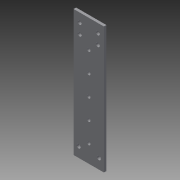
# Autodesk Inventor part: Support for 9-16 Piston
Saved by Autodesk Inventor 2014 (Build 180170000, 170)
## iProperties
Created: 2014-01-07
Part Number: Support for 9-16 Piston
Material: Generic
Document SubType Name: Modeling
Designer: Michael
Density: 1 g/cm^3
Appearance: Default
Author: Michael
Autodesk Inventor part; units mm, degrees
ref_plane "YZ Plane" through (0, 0, 0) normal (1, 0, 0) x (0, 1, 0)
ref_plane "XZ Plane" through (0, 0, 0) normal (0, 1, 0) x (-1, 0, 0)
ref_plane "XY Plane" through (0, 0, 0) normal (0, 0, 1) x (1, 0, 0)
sketch "Sketch1" plane through (0, 0, 0) normal (0, 0, 1) x (1, 0, 0)
  line L0 (38.1, 0) -> (38.1, -3.175)
  line L1 (0, 0) -> (38.1, 0)
  line L2 (38.1, 0) -> (38.1, -158.75)
  line L3 (38.1, -158.75) -> (0, -158.75)
  line L4 (0, -158.75) -> (0, 0)
  circle A0 centre (6.35, -146.05) radius 2.4384
  line L5 (19.05, -158.75) -> (19.05, 0) construction
  circle A1 centre (31.75, -146.05) radius 2.4384
  circle A2 centre (7.6581, -23.6982) radius 2.4384
  circle A3 centre (7.6581, -10.9982) radius 2.4384
  circle A4 centre (30.4419, -10.9982) radius 2.4384
  circle A5 centre (30.4419, -23.6982) radius 2.4384
  line L6 (7.6581, -10.9982) -> (7.6581, -23.6982) construction
  line L7 (31.75, -136.525) -> (6.35, -136.525) construction
  line L8 (6.35, -136.525) -> (6.35, -34.925) construction
  line L9 (6.35, -34.925) -> (31.75, -34.925) construction
  line L10 (31.75, -34.925) -> (31.75, -136.525) construction
  circle A6 centre (19.05, -34.925) radius 2.0828
  circle A7 centre (19.05, -60.325) radius 2.0828
  circle A8 centre (19.05, -85.725) radius 2.0828
  circle A9 centre (19.05, -111.125) radius 2.0828
  circle A10 centre (19.05, -136.525) radius 2.0828
  dimension "d0" = 4.8768
  dimension "d1" = 158.75
  dimension "d2" = 12.7
  dimension "d3" = 12.7
  dimension "d4" = 12.7
  dimension "d5" = 11.3919
  dimension "d6" = 122.3518
  dimension "d7" = 38.1
  dimension "d8" = 25.4
  dimension "d9" = 34.925
  dimension "d10" = 101.6
  dimension "d11" = 4.1656
  dimension "d14" = 25.4
  constraints: 22 end point, 11 centre point, 4 parallel, 3 midpoint, 3 symmetric about line, 3 vertical, 2 equal radius, 2 horizontal, 2 perpendicular, 1 coincident, 1 collinear, 1 point on line, 12 other
  measures "d0" diameter of A0
  measures "d1" distance of L4.start L4.end
  measures "d2" distance from line of L5 A0.centre
  measures "d3" distance from line of L3 A0.centre
  measures "d4" distance of L6.end L6.start
  measures "d5" distance from line of L5 L6.end
  measures "d6" vertical distance of L6.end A0.centre
  measures "d7" distance of L4.end L2.start
  measures "d8" distance of L8.end L9.end
  measures "d9" distance between parallel lines of L1 L9
  measures "d10" distance of L9.end L7.start
  measures "d11" diameter of A6
  measures "d14" distance of A6.centre A7.centre
extrude "Extrusion1" add sketch "Sketch1" along normal blind 3.175
body "Solid1"
